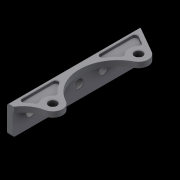
# Autodesk Inventor part: SpineMiddleCover
Saved by Autodesk Inventor 2015 (Build 190159000, 159)
## iProperties
Created: 2015-01-07
Part Number: SpineMiddleCover
Material: Generic
Document SubType Name: Modeling
Designer: Val
Density: 1 g/cm^3
Appearance: Default
Mass: 1.14982 g
Surface Area: 17.1858 cm^2
Volume: 1.14982 cm^3
Author: Val
Autodesk Inventor part; units mm, degrees
ref_plane "YZ Plane" through (0, 0, 0) normal (1, 0, 0) x (0, 1, 0)
ref_plane "XZ Plane" through (0, 0, 0) normal (0, 1, 0) x (-1, 0, 0)
ref_plane "XY Plane" through (0, 0, 0) normal (0, 0, 1) x (1, 0, 0)
sketch "TopProfile" plane through (0, 0, 0) normal (0, 0, 1) x (1, 0, 0)
  circle A0 centre (0, 15.5) radius 3.5
  circle A1 centre (0, -15.5) radius 3.5
  line L0 (1.75, 18.5311) -> (-8.5, 24.4489)
  line L1 (-8.5, -23.5511) -> (-8.5, 24.4489)
  arc A2 (1.6248, 12.4) -> (1.6248, -12.4) centre (8.124, 0) ccw
  line L2 (-8.5, -23.5511) -> (-6, -23.5511)
  arc A3 (0.6576, -18.9377) -> (-6, -23.5511) centre (2.5365, -28.7596) ccw
  line L3 (0, -15.5) -> (0, 15.5) construction
  circle A4 centre (0, 15.5) radius 1.5
  circle A5 centre (0, -15.5) radius 1.5
  point P0 (0, 0)
  point P1 (0, 0)
  dimension "d1" = 7
  dimension "d3" = 2.5
  dimension "d4" = 60
  dimension "d5" = 48
  dimension "d6" = 14
  dimension "d7" = 31
  dimension "d9" = 8.5
  dimension "d10" = 3
  dimension "d12" = 10
  constraints: 8 end point, 8 point on circle, 6 centre point, 4 tangent, 3 coincident, 2 equal radius, 1 midpoint, 1 parallel, 1 perpendicular, 1 vertical
  measures "d1" diameter of A0
  measures "d3" distance of L1.start L2.end
  measures "d4" angle of L0 L1
  measures "d5" distance of L1.start L0.end
  measures "d6" radius of A2
  measures "d7" distance of L3.start L3.end
  measures "d9" distance between parallel lines of L1 L3
  measures "d10" diameter of A4
  measures "d12" radius of A3
extrude "TopProfileFeature" add sketch "TopProfile" along normal blind 10
sketch "FrontProfile" plane through (-8.5, -23.5511, 0) normal (0, -1, 0) x (1, 0, 0)
  line L0 (0, 0) -> (0, 10) construction
  line L1 (0, 10) -> (2.5, 10) projected
  line L2 (12, 0) -> (12, 10) construction
  line L3 (0, 10) -> (12, 10)
  line L4 (12, 10) -> (9.1576, 10) projected
  line L5 (0, 10) -> (0, 0)
  line L6 (0, 0) -> (2, 0)
  line L7 (2, 0) -> (2, 8)
  line L8 (2, 8) -> (12, 8)
  line L9 (12, 10) -> (12, 8)
  line L10 (0, 0) -> (2.5, 0) projected
  point P0 (10.1248, 10)
  dimension "d16" = 2
  dimension "d45" = 2
  constraints: 12 end point, 4 collinear, 2 perpendicular, 1 point on line, 1 vertical
  measures "d16" distance between parallel lines of L3 L8
  measures "d45" distance between parallel lines of L0 L7
extrude "FrontProfileFeature" cut sketch "FrontProfile" against normal through all keep common part
fillet "SideFilletFeature" radius 1 1 edges at (-8.5, 0.4489, 10)
sketch "Sinks" plane through (0, 0, 10) normal (0, 0, 1) x (1, 0, 0)
  circle A0 centre (0, 15.5) radius 1.5 construction
  circle A1 centre (0, -15.5) radius 1.5 construction
  circle A2 centre (0, 15.5) radius 3.5
  circle A3 centre (0, -15.5) radius 3.5
  line L0 (-1.4875, 18.6682) -> (-7, 21.8509)
  line L1 (-7, 21.8509) -> (-7, 4)
  arc A4 (-1.3472, 12.2697) -> (-6.8509, 4) centre (8.124, 0) ccw
  line L2 (1.75, 18.5311) -> (-7.5, 23.8716) construction
  line L3 (-8.5, 24.4489) -> (-8.5, -23.5511) construction
  arc A5 (1.6248, 12.4) -> (1.6248, -12.4) centre (8.124, 0) ccw construction
  line L4 (-7, -4) -> (-7, -22.3326)
  arc A6 (-6.8509, -4) -> (-1.3472, -12.2697) centre (8.124, 0) ccw
  arc A7 (-2.1532, -18.2593) -> (-7, -22.3326) centre (2.5365, -28.7596) ccw
  arc A8 (0.6576, -18.9377) -> (-6, -23.5511) centre (2.5365, -28.7596) ccw construction
  line L5 (-7, 4) -> (-6.8509, 4)
  line L6 (-6.8509, -4) -> (-7, -4)
  arc A9 (1.6248, 12.4) -> (1.6248, -12.4) centre (8.124, 0) ccw construction
  line L7 (-5.876, 0) -> (-8.5, 0) construction
  line L8 (-8.5, 24.4489) -> (-8.5, -23.5511) construction
  point P0 (0, 0)
  dimension "d20" = 1.5
  dimension "d21" = 1.5
  dimension "d22" = 1.5
  dimension "d23" = 1.5
  dimension "d24" = 1.5
  dimension "d50" = 4
  dimension "d51" = 4
  constraints: 14 point on circle, 12 end point, 5 centre point, 3 concentric, 2 coincident, 2 parallel, 2 perpendicular, 1 collinear, 1 horizontal, 1 point on line, 1 vertical
  measures "d20" distance between parallel lines of L2 L0
  measures "d21" radial gap between concentric circles of A5 A4
  measures "d22" distance between parallel lines of L3 L1
  measures "d23" radial gap between concentric circles of A5 A6
  measures "d24" radial gap between concentric circles of A8 A7
  measures "d50" distance between parallel lines of L7 L5
  measures "d51" distance between parallel lines of L7 L6
extrude "SinksFeature" cut sketch "Sinks" against normal blind 1 contours A2 A4 L5 L1 L0 | A3 A7 L4 L6 A6
fillet "SinkFilletsFeature" radius 1 10 edges at (-7, 21.8509, 9.5) (-7, 4, 9.5) (-1.3472, 12.2697, 9.5) (-1.4875, 18.6682, 9.5) (-7, -22.3326, 9.5) (-7, -4, 9.5) (-1.3472, -12.2697, 9.5) (-2.1532, -18.2593, 9.5) (-6.8509, 4, 9.5) (-6.8509, -4, 9.5)
sketch "SideHoles" plane through (-8.5, -23.5511, 0) normal (-1, 0, 0) x (0, 0, 1)
  line L0 (10, 0) -> (10, 47.4226) construction
  line L1 (0, 48) -> (9, 48) construction
  circle A0 centre (5, 41.5) radius 1.75
  line L2 (5, 41.5) -> (5, 6.5) construction
  circle A1 centre (5, 24) radius 1.75
  circle A2 centre (5, 6.5) radius 1.75
  line L3 (5, 24) -> (0, 24) construction
  circle A3 centre (5, 15.25) radius 1.75
  circle A4 centre (5, 32.75) radius 1.75
  line L4 (0, 48) -> (0, 0) construction
  line L5 (8, 0) -> (0, 0) projected
  dimension "d28" = 3.5
  dimension "d30" = 5
  dimension "d33" = 35
  dimension "d43" = 8.75
  dimension "d44" = 8.75
  dimension "d46" = 5
  dimension "d47" = 6.5
  dimension "d48" = 6.5
  constraints: 5 centre point, 4 end point, 4 equal radius, 2 midpoint, 2 point on line, 1 coincident, 1 horizontal, 1 vertical
  measures "d28" diameter of A0
  measures "d30" distance between parallel lines of L0 L2
  measures "d33" distance of L2.start L2.end
  measures "d43" distance of L3.start A3.centre
  measures "d44" distance of A4.centre L3.start
  measures "d46" distance between parallel lines of L4 L2
  measures "d47" distance from line of L1 L2.start
  measures "d48" distance from line of L5 L2.end
hole "SideHolesFeature" at (-8.5, 17.9489, 5) at (-8.5, 0.4489, 5) at (-8.5, -17.0511, 5) at (-8.5, 9.1989, 5) at (-8.5, -8.3011, 5) direction (1, 0, 0) diameter 3 end through all
fillet "BottomCornerFilletsFeature" radius 1 2 edges at (-7.5, -23.5511, 0) (-7.5, 23.8716, 0)
equation "\"d21\" = d20"
equation "\"d22\" = d20"
equation "\"d23\" = d20"
equation "\"d24\" = d20"
equation "\"d51\" = d50"
equation "\"d30\" = 0.5 * d29"
equation "\"d43\" = 0.25 * d33"
equation "\"d44\" = d43"
equation "\"d47\" = d48"
equation "\"d29\" = 10"
